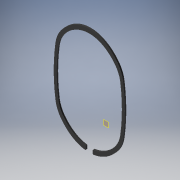
# Autodesk Inventor part: FrameRim
Saved by Autodesk Inventor 2018 (Build 220112000, 112)
## iProperties
Created: 2018-06-05
Part Number: FrameRim
Material: Generic
Document SubType Name: Modeling
Designer: reide
Density: 1 g/cm^3
Appearance: Default
Author: reide
Autodesk Inventor part; units mm, degrees
ref_plane "YZ Plane" through (0, 0, 0) normal (1, 0, 0) x (0, 1, 0)
ref_plane "XZ Plane" through (0, 0, 0) normal (0, 1, 0) x (-1, 0, 0)
ref_plane "XY Plane" through (0, 0, 0) normal (0, 0, 1) x (1, 0, 0)
ref_plane "Work Plane2" through (0, 0, 0) normal (0, 0, 1) x (1, 0, 0)
sketch "Sketch1" plane through (0, 0, 0) normal (0, 0, 1) x (1, 0, 0)
  circle A0 centre (-192.358, 126.614) radius 1.75 projected
  arc A1 (81.2372, 206.8201) -> (56.4499, 266.1206) centre (-44.5185, 189.0856) ccw
  ellipse E0 centre (-68.0111, 96.3387) end of major axis (-68.0111, -141.4053) minor radius 177.8 (56.4499, 266.1206) -> (-192.4721, 266.1206) ccw
  arc A2 (-192.4721, 266.1206) -> (-217.2594, 206.8201) centre (-91.5037, 189.0856) ccw
  arc A3 (-217.2594, 206.8201) -> (-217.2594, -14.1426) centre (566.1677, 96.3387) ccw
  arc A4 (-217.2594, -14.1426) -> (-192.4721, -73.4431) centre (-91.5037, 3.5918) ccw
  ellipse E1 centre (-68.0111, 96.3387) end of major axis (-68.0111, -141.4053) minor radius 177.8 (-192.4721, -73.4431) -> (56.4499, -73.4431) ccw
  arc A5 (56.4499, -73.4431) -> (81.2372, -14.1426) centre (-44.5185, 3.5918) ccw
  arc A6 (81.2372, -14.1426) -> (81.2372, 206.8201) centre (-702.1899, 96.3387) ccw
  constraints: 12 point on circle, 6 centre point, 8 other
extrude "Extrusion1" add sketch "Sketch1" along normal blind 6.35 contours A0 | A6 A5 E1 A4 A3 A2 E0 A1
sketch "Sketch2" plane through (0, 0, 6.35) normal (0, 0, 1) x (1, 0, 0)
  circle A0 centre (-183.032, 124.3433) radius 1.6187
  arc A1 (70.0436, 198.534) -> (47.1154, 253.3869) centre (-46.2804, 182.1296) ccw
  ellipse E0 centre (-68.0111, 96.3387) end of major axis (-68.0111, -123.5745) minor radius 164.465 (47.1154, 253.3869) -> (-183.1375, 253.3869) ccw
  arc A2 (-183.1375, 253.3869) -> (-206.0658, 198.534) centre (-89.7418, 182.1296) ccw
  arc A3 (-206.0658, 198.534) -> (-206.0658, -5.8565) centre (518.6043, 96.3387) ccw
  arc A4 (-206.0658, -5.8565) -> (-183.1375, -60.7095) centre (-89.7418, 10.5478) ccw
  ellipse E1 centre (-68.0111, 96.3387) end of major axis (-68.0111, -123.5745) minor radius 164.465 (-183.1375, -60.7095) -> (47.1154, -60.7095) ccw
  arc A5 (47.1154, -60.7095) -> (70.0436, -5.8565) centre (-46.2804, 10.5478) ccw
  arc A6 (70.0436, -5.8565) -> (70.0436, 198.534) centre (-654.6265, 96.3387) ccw
  point P0 (0, 0)
  constraints: 12 point on circle, 7 centre point, 8 other
extrude "Extrusion2" cut sketch "Sketch2" against normal blind 6.35 contours A0 | A6 A5 E1 A4 A3 A2 E0 A1
sketch "Sketch3" plane through (0, 0, 6.35) normal (0, 0, 1) x (1, 0, 0)
  circle A0 centre (-196.3999, 49.2593) radius 1.75 projected
  circle A1 centre (-190.196, 38.5473) radius 1.75 projected
  circle A2 centre (-167.6724, 59.9713) radius 1.75 projected
  circle A3 centre (-167.6724, 38.5473) radius 1.75 projected
  circle A4 centre (-161.4685, 49.2593) radius 1.75 projected
  circle A5 centre (54.1738, 59.9713) radius 1.75 projected
  circle A6 centre (60.3777, 49.2593) radius 1.75 projected
  circle A7 centre (25.4463, 29.0473) radius 1.75 projected
  circle A8 centre (25.4463, 49.2593) radius 1.75 projected
  circle A9 centre (25.4463, 69.4713) radius 1.75 projected
  circle A10 centre (31.6502, 59.9713) radius 1.75 projected
  circle A11 centre (31.6502, 38.5473) radius 1.75 projected
  circle A12 centre (54.1738, 38.5473) radius 1.75 projected
  circle A13 centre (60.3777, 29.0473) radius 1.75 projected
  circle A14 centre (60.3777, 69.4713) radius 1.75 projected
  circle A15 centre (-161.4685, 29.0473) radius 1.75 projected
  circle A16 centre (-190.196, 59.9713) radius 1.75 projected
  circle A17 centre (-161.4685, 69.4713) radius 1.75 projected
  circle A18 centre (-196.3999, 29.0473) radius 1.75 projected
  circle A19 centre (-196.3999, 69.4713) radius 1.75 projected
  circle A20 centre (-192.358, 126.614) radius 1.75 projected
  circle A21 centre (-166.2135, 137.114) radius 1.75 projected
  circle A22 centre (-151.3535, 137.114) radius 1.75 projected
  circle A23 centre (56.3358, 169.2663) radius 1.75 projected
  circle A24 centre (30.1913, 137.114) radius 1.75 projected
  circle A25 centre (30.1913, 169.114) radius 1.75 projected
  circle A26 centre (15.3313, 169.114) radius 1.75 projected
  circle A27 centre (15.3313, 137.114) radius 1.75 projected
  circle A28 centre (56.3358, 126.614) radius 1.75 projected
  circle A29 centre (-166.2135, 169.114) radius 1.75 projected
  circle A30 centre (-192.358, 169.2663) radius 1.75 projected
  circle A31 centre (-151.3535, 169.114) radius 1.75 projected
  circle A32 centre (-125.2039, 71.3387) radius 1.75 projected
  circle A33 centre (-10.8188, 71.3387) radius 1.75 projected
  circle A34 centre (-125.2036, 96.9184) radius 1.75 projected
  circle A35 centre (-10.8185, 96.9184) radius 1.75 projected
  circle A36 centre (-10.8187, 86.9184) radius 1.75 projected
  circle A37 centre (-125.2035, 86.9184) radius 1.75 projected
  circle A38 centre (-10.8188, 61.3387) radius 1.75 projected
  circle A39 centre (-125.2039, 61.3387) radius 1.75 projected
  circle A40 centre (-68.6105, -28.321) radius 1.63 projected
  arc A41 (-88.5111, 275.0837) -> (-92.5111, 275.0837) centre (-90.5111, 275.0837) ccw projected
  line L0 (-88.5111, 275.0837) -> (-88.5111, 230.0837) projected
  arc A42 (-92.5111, 230.0837) -> (-88.5111, 230.0837) centre (-90.5111, 230.0837) ccw projected
  line L1 (-92.5111, 230.0837) -> (-92.5111, 275.0837) projected
  arc A43 (-43.5111, 275.0837) -> (-47.5111, 275.0837) centre (-45.5111, 275.0837) ccw projected
  line L2 (-43.5111, 275.0837) -> (-43.5111, 230.0837) projected
  arc A44 (-47.5111, 230.0837) -> (-43.5111, 230.0837) centre (-45.5111, 230.0837) ccw projected
  line L3 (-47.5111, 230.0837) -> (-47.5111, 275.0837) projected
  circle A45 centre (-6.132, -79.3472) radius 1.25 projected
  circle A46 centre (-145.3842, 185.8247) radius 1.5 projected
  circle A47 centre (-153.8932, -1.3222) radius 1.5 projected
  circle A48 centre (-145.3842, -79.3472) radius 1.5 projected
  circle A49 centre (-129.8902, 6.8528) radius 1.5 projected
  circle A50 centre (-116.3012, -71.1722) radius 1.5 projected
  circle A51 centre (-129.8902, 272.0247) radius 1.5 projected
  circle A52 centre (-129.8902, 185.8247) radius 1.5 projected
  circle A53 centre (-116.3012, 263.8497) radius 1.5 projected
  circle A54 centre (17.871, -71.1722) radius 1.5 projected
  circle A55 centre (-6.132, 6.8528) radius 1.5 projected
  circle A56 centre (-19.721, -1.3222) radius 1.5 projected
  circle A57 centre (17.871, 263.8497) radius 1.5 projected
  circle A58 centre (9.362, 272.0247) radius 1.5 projected
  circle A59 centre (9.362, 185.8247) radius 1.5 projected
  circle A60 centre (-19.721, 193.9997) radius 1.5 projected
  circle A61 centre (-19.721, 263.8497) radius 1.5 projected
  circle A62 centre (-6.132, 185.8247) radius 1.5 projected
  circle A63 centre (-6.132, 272.0247) radius 1.5 projected
  circle A64 centre (17.871, 193.9997) radius 1.5 projected
  circle A65 centre (-19.721, -71.1722) radius 1.5 projected
  circle A66 centre (9.362, -79.3472) radius 1.5 projected
  circle A67 centre (9.362, 6.8528) radius 1.5 projected
  circle A68 centre (17.871, -1.3222) radius 1.5 projected
  circle A69 centre (-116.3012, 193.9997) radius 1.5 projected
  circle A70 centre (-153.8932, 193.9997) radius 1.5 projected
  circle A71 centre (-153.8932, 263.8497) radius 1.5 projected
  circle A72 centre (-145.3842, 6.8528) radius 1.5 projected
  circle A73 centre (-129.8902, -79.3472) radius 1.5 projected
  circle A74 centre (-153.8932, -71.1722) radius 1.5 projected
  circle A75 centre (-116.3012, -1.3222) radius 1.5 projected
  circle A76 centre (-145.3842, 272.0247) radius 1.5 projected
  arc A77 (81.2372, 206.8201) -> (56.4499, 266.1206) centre (-44.5185, 189.0856) ccw projected
  ellipse E0 centre (-68.0111, 96.3387) end of major axis (-68.0111, -141.4053) minor radius 177.8 (56.4499, 266.1206) -> (-192.4721, 266.1206) ccw projected
  arc A78 (-192.4721, 266.1206) -> (-217.2594, 206.8201) centre (-91.5037, 189.0856) ccw projected
  arc A79 (-217.2594, 206.8201) -> (-217.2594, -14.1426) centre (566.1677, 96.3387) ccw projected
  arc A80 (-217.2594, -14.1426) -> (-192.4721, -73.4431) centre (-91.5037, 3.5918) ccw projected
  ellipse E1 centre (-68.0111, 96.3387) end of major axis (-68.0111, -141.4053) minor radius 177.8 (-192.4721, -73.4431) -> (56.4499, -73.4431) ccw projected
  arc A81 (56.4499, -73.4431) -> (81.2372, -14.1426) centre (-44.5185, 3.5918) ccw projected
  arc A82 (81.2372, -14.1426) -> (81.2372, 206.8201) centre (-702.1899, 96.3387) ccw projected
  circle A83 centre (-35.6216, 248.9087) radius 1.25 projected
  circle A84 centre (-100.4006, 318.7587) radius 1.25 projected
  circle A85 centre (-100.4006, 248.9087) radius 1.25 projected
  circle A86 centre (-35.6216, 318.7587) radius 1.25 projected
  circle A87 centre (-56.9111, -118.4053) radius 1.5 projected
  circle A88 centre (-79.1111, -118.4053) radius 1.5 projected
  circle A89 centre (-58.7361, -128.5803) radius 1.5 projected
  circle A90 centre (-61.0891, -46.904) radius 1.5 projected
  circle A91 centre (-53.9141, -54.079) radius 1.5 projected
  circle A92 centre (-92.2681, -54.079) radius 1.5 projected
  circle A93 centre (-85.0931, -46.904) radius 1.5 projected
  circle A94 centre (-77.2861, -128.5803) radius 1.5 projected
  circle A95 centre (-79.1111, -110.4053) radius 1.5 projected
  circle A96 centre (-56.9111, -110.4053) radius 1.5 projected
  line L4 (-82.971, -17.5241) -> (-82.971, 43.3967) projected
  line L5 (-82.971, 43.3967) -> (-52.491, 43.3967) projected
  line L6 (-52.491, 43.3967) -> (-52.491, -17.5241) projected
  line L7 (-52.491, -17.5241) -> (-82.971, -17.5241) projected
  circle A97 centre (-68.0111, 137.616) radius 35 projected
  line L8 (-123.7158, 171.3631) -> (-119.7158, 171.3631) projected
  arc A98 (-119.7158, 168.3632) -> (-119.7158, 171.3631) centre (-119.7158, 169.8631) ccw projected
  line L9 (-119.7158, 168.3632) -> (-123.7158, 168.3632) projected
  arc A99 (-123.7158, 171.3631) -> (-123.7158, 168.3632) centre (-123.7158, 169.8631) ccw projected
  line L10 (-123.6698, 106.6744) -> (-119.6698, 106.6744) projected
  arc A100 (-119.6698, 103.6746) -> (-119.6698, 106.6744) centre (-119.6698, 105.1745) ccw projected
  line L11 (-119.6698, 103.6746) -> (-123.6698, 103.6746) projected
  arc A101 (-123.6698, 106.6744) -> (-123.6698, 103.6746) centre (-123.6698, 105.1745) ccw projected
  line L12 (-9.1669, 171.4444) -> (-5.1669, 171.4444) projected
  arc A102 (-5.1669, 168.4446) -> (-5.1669, 171.4444) centre (-5.1669, 169.9445) ccw projected
  line L13 (-5.1669, 168.4446) -> (-9.1669, 168.4446) projected
  arc A103 (-9.1669, 171.4444) -> (-9.1669, 168.4446) centre (-9.1669, 169.9445) ccw projected
  line L14 (-5.1669, 103.6742) -> (-9.1669, 103.6742) projected
  arc A104 (-9.1669, 106.6741) -> (-9.1669, 103.6742) centre (-9.1669, 105.1742) ccw projected
  line L15 (-9.1669, 106.6741) -> (-5.1669, 106.6741) projected
  arc A105 (-5.1669, 103.6742) -> (-5.1669, 106.6741) centre (-5.1669, 105.1742) ccw projected
  arc A106 (-34.0816, 86.6493) -> (-37.0792, 86.6494) centre (-35.5804, 86.6492) ccw projected
  line L16 (-34.0816, 86.6493) -> (-34.0814, 82.6493) projected
  arc A107 (-37.0794, 82.6493) -> (-34.0814, 82.6493) centre (-35.5804, 82.6492) ccw projected
  line L17 (-37.0794, 82.6493) -> (-37.0792, 86.6494) projected
  arc A108 (-34.0865, 201.0395) -> (-37.0841, 201.0395) centre (-35.5853, 201.0395) ccw projected
  line L18 (-34.0865, 201.0395) -> (-34.0863, 197.0396) projected
  arc A109 (-37.0843, 197.0395) -> (-34.0863, 197.0396) centre (-35.5853, 197.0395) ccw projected
  line L19 (-37.0843, 197.0395) -> (-37.0841, 201.0395) projected
  arc A110 (-34.0812, 78.9993) -> (-37.0788, 78.9992) centre (-35.58, 78.9992) ccw projected
  line L20 (-34.0812, 78.9993) -> (-34.081, 74.9993) projected
  arc A111 (-37.079, 74.9993) -> (-34.081, 74.9993) centre (-35.58, 74.9992) ccw projected
  line L21 (-37.079, 74.9993) -> (-37.0788, 78.9992) projected
  arc A112 (-98.9325, 193.3865) -> (-101.9301, 193.3866) centre (-100.4313, 193.3865) ccw projected
  line L22 (-98.9325, 193.3865) -> (-98.9323, 189.3866) projected
  arc A113 (-101.9303, 189.3866) -> (-98.9323, 189.3866) centre (-100.4313, 189.3865) ccw projected
  line L23 (-101.9303, 189.3866) -> (-101.9301, 193.3866) projected
  circle A114 centre (-95.163, -4.4165) radius 1.25 projected
  circle A115 centre (-36.616, 37.0467) radius 1.25 projected
  circle A116 centre (-46.141, -14.3491) radius 1.25 projected
  circle A117 centre (-36.616, -11.1741) radius 1.25 projected
  circle A118 centre (-36.616, 12.9421) radius 1.25 projected
  circle A119 centre (-46.141, 40.2217) radius 1.25 projected
  circle A120 centre (-95.163, 40.4375) radius 1.25 projected
  arc A121 (-98.8512, 78.9533) -> (-101.8488, 78.9533) centre (-100.35, 78.9533) ccw projected
  line L24 (-98.8512, 78.9533) -> (-98.851, 74.9533) projected
  arc A122 (-101.849, 74.9533) -> (-98.851, 74.9533) centre (-100.35, 74.9533) ccw projected
  line L25 (-101.849, 74.9533) -> (-101.8488, 78.9533) projected
  line L26 (-34.0865, 193.3895) -> (-34.0863, 189.3896) projected
  arc A123 (-37.0843, 189.3896) -> (-34.0863, 189.3896) centre (-35.5853, 189.3895) ccw projected
  line L27 (-37.0843, 189.3896) -> (-37.0841, 193.3896) projected
  arc A124 (-34.0865, 193.3895) -> (-37.0841, 193.3896) centre (-35.5853, 193.3895) ccw projected
  arc A125 (-98.9379, 201.0395) -> (-101.9362, 200.9947) centre (-100.4367, 200.9934) ccw projected
  line L28 (-98.9379, 201.0395) -> (-98.9377, 196.9935) projected
  arc A126 (-101.9357, 196.9932) -> (-98.9377, 196.9935) centre (-100.4367, 196.9934) ccw projected
  line L29 (-101.9357, 196.9932) -> (-101.9362, 200.9947) projected
  arc A127 (-98.8567, 86.6032) -> (-101.8543, 86.6033) centre (-100.3555, 86.6032) ccw projected
  line L30 (-98.8567, 86.6032) -> (-98.8565, 82.6033) projected
  arc A128 (-101.8544, 82.6033) -> (-98.8565, 82.6033) centre (-100.3555, 82.6032) ccw projected
  line L31 (-101.8544, 82.6033) -> (-101.8543, 86.6033) projected
  line L32 (-16.8169, 106.6744) -> (-12.8169, 106.6744) projected
  arc A129 (-12.8169, 103.6746) -> (-12.8169, 106.6744) centre (-12.8169, 105.1745) ccw projected
  line L33 (-12.8169, 103.6746) -> (-16.8169, 103.6746) projected
  arc A130 (-16.8169, 106.6744) -> (-16.8169, 103.6746) centre (-16.8169, 105.1745) ccw projected
  line L34 (-16.8629, 171.439) -> (-12.8629, 171.439) projected
  arc A131 (-12.8629, 168.4391) -> (-12.8629, 171.439) centre (-12.8629, 169.9391) ccw projected
  line L35 (-12.8629, 168.4391) -> (-16.8629, 168.4391) projected
  arc A132 (-16.8629, 171.439) -> (-16.8629, 168.4391) centre (-16.8629, 169.9391) ccw projected
  line L36 (-131.3198, 106.6744) -> (-127.3198, 106.6744) projected
  arc A133 (-127.3198, 103.6746) -> (-127.3198, 106.6744) centre (-127.3198, 105.1745) ccw projected
  line L37 (-127.3198, 103.6746) -> (-131.3198, 103.6746) projected
  arc A134 (-131.3198, 106.6744) -> (-131.3198, 103.6746) centre (-131.3198, 105.1745) ccw projected
  line L38 (-131.3658, 171.3576) -> (-127.3658, 171.3576) projected
  arc A135 (-127.3658, 168.3578) -> (-127.3658, 171.3576) centre (-127.3658, 169.8577) ccw projected
  line L39 (-127.3658, 168.3578) -> (-131.3658, 168.3578) projected
  arc A136 (-131.3658, 171.3576) -> (-131.3658, 168.3578) centre (-131.3658, 169.8577) ccw projected
  line L40 (-84.1111, -106.4053) -> (-84.1111, -139.5398) projected
  line L41 (-51.9111, -139.5398) -> (-51.9111, -106.4053) projected
  line L42 (-84.1111, -122.3838) -> (-51.9111, -122.3838)
  line L43 (-51.9111, -122.3838) -> (-51.9111, -147.7518)
  line L44 (-51.9111, -147.7518) -> (-84.1111, -147.7518)
  line L45 (-84.1111, -147.7518) -> (-84.1111, -122.3838)
  point P0 (0, 0)
  constraints: 8 end point, 2 parallel, 1 horizontal, 1 perpendicular, 1 point on line, 2 other
extrude "Extrusion3" cut sketch "Sketch3" against normal blind 6.35 contours L43 L44 L45 E1 | E1 L45 L40 L42 L41 L43 | A89 | A94
fillet "Fillet1" radius 2 4 edges at (-84.1111, -140.4286, 3.175) (-51.9111, -140.4286, 3.175) (-84.1111, -122.5182, 3.175) (-51.9111, -122.5182, 3.175)
body "Solid1"
